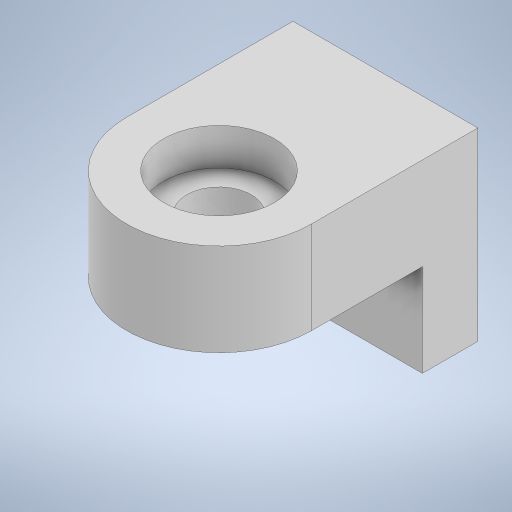
# Autodesk Inventor part: podpora_lewa
Saved by Autodesk Inventor 2023 (Build 270158000, 158)
## iProperties
Created: 2024-05-21
Part Number: podpora_lewa
Material: Ogólny
Document SubType Name: Modeling
Designer: kamil
Density: 1 g/cm^3
Appearance: Domyślna
Author: kamil
Autodesk Inventor part; units mm, degrees
ref_plane "YZ Plane" through (0, 0, 0) normal (1, 0, 0) x (0, 1, 0)
ref_plane "XZ Plane" through (0, 0, 0) normal (0, 1, 0) x (-1, 0, 0)
ref_plane "XY Plane" through (0, 0, 0) normal (0, 0, 1) x (1, 0, 0)
sketch "Szkic1" plane through (0, 0, 0) normal (0, 1, 0) x (-1, 0, 0)
  circle A0 centre (0, 0) radius 1.5
  circle A1 centre (0, 0) radius 5
  line L0 (5, 0) -> (-5, 0)
  line L1 (-5, 0) -> (-5, -6)
  line L2 (-5, -6) -> (5, -6)
  line L3 (5, -6) -> (5, 0)
  dimension "d1" = 10
  dimension "d0" = 3
  dimension "d2" = 6
  constraints: 8 end point, 2 coincident, 2 parallel, 1 centre point, 1 horizontal, 1 perpendicular, 3 other
  measures "d0" diameter of A0
  measures "d2" distance of L1.end L0.end
extrude "Wyciągnięcie proste1" add sketch "Szkic1" along normal blind 5
sketch "Szkic2" plane through (5, 0, -6) normal (0, 0, -1) x (-1, 0, 0)
  line L0 (0, 0) -> (10, 0) projected
  line L1 (10, 0) -> (10, 5) projected
  line L2 (0, 5) -> (10, 5) projected
  line L3 (0, 0) -> (0, 5) projected
  line L4 (0, 5) -> (10, 5)
  line L5 (10, 5) -> (10, -5)
  line L6 (10, -5) -> (0, -5)
  line L7 (0, -5) -> (0, 5)
  point P0 (5, 0)
  dimension "d5" = 5
  constraints: 8 end point, 2 parallel, 1 horizontal, 1 perpendicular
  measures "d5" distance between parallel lines of L6 L0
extrude "Wyciągnięcie proste2" add sketch "Szkic2" along normal blind 3
sketch "Szkic3" plane through (0, 5, 0) normal (0, 1, 0) x (1, 0, 0)
  point P0 (0, 0)
  point P1 (0, 0)
  constraints: 1 coincident
hole "Otwór1" at (0, 5, 0) direction (0, -1, 0) diameter 3.5 end through all counterbore diameter 6 counterbore depth 2
